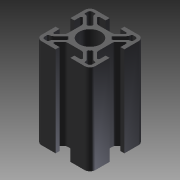
# Autodesk Inventor part: MayTec 1.11.030030.43SP_Profile 30x30. 4F, SP_50_Detail_(0;0,0,0)
Saved by Autodesk Inventor 2011 SP1 (Build 150282100, 282)
## iProperties
Created: 2018-01-06
Part Number: MayTec 1.11.030030.43SP_Profile 30x30. 4F, SP_50_Detail_(0;0,0,0)
Catalog Web Link: www.cadenas.de
Description: 1.11.030030.43SP-Profile 30x30. 4F, SP
Vendor: MAYTEC
Document SubType Name: Modeling
Designer: psAdmin
Manufacturer: MAYTEC
Mass: 18.6034 g
Surface Area: 180.256 cm^2
Volume: 18.6034 cm^3
Density: 1 g/cm^3
Category: PARTsolutions
Company: MAYTEC
Title: MayTec 1.11.030030.43SP_Profile 30x30. 4F, SP_50_Detail_(0;0,0,0)
Author: Cadenas PARTsolutions
Comments: Profile 30x30. 4F, SP
PSOL_IDENT_0: {$CADENAS_DATA\23d-libs\maytec\maytec_3d\profile\profilgruppe_30\30x30\1.11.030030.43sp.prj},299 {VT
PSOL_IDENT_1: YP=3D},{NB=MayTec 1.11.030030.43SP_Profile 30x30. 4F, SP_50_Detail_(0;0,0,0)},{LINA=MayTec 1.11.0300
PSOL_IDENT_2: 30.43SP_Profile 30x30. 4F, SP_50_Detail_(0;0,0,0)},{NN=1.11.030030.43SP},{DATE=09.02.2017 10:28:55},
PSOL_IDENT_3: {GEOMDATE=07.02.2017 11:09:15},{VERSION=},{LINEID=10},{LINESUBID=-1},{WBVAR=L,SAX,SAY,EAX,EAY}  {NB=
PSOL_IDENT_4: MayTec 1.11.030030.43SP_Profile 30x30. 4F, SP_50_Detail_(0;0,0,0)},{LINA=MayTec 1.11.030030.43SP_Pro
PSOL_IDENT_5: file 30x30. 4F, SP_50_Detail_(0;0,0,0)},{KT=DUMMY},{PARTNR=1.11.030030.43SP},{DESCRIPTION=Profil 30x
PSOL_IDENT_6: 30, 4F, SP},{L=50.00},{DETAIL=Detail},{D=1},{XTRANS=Profile 30x30. 4F, SP},{SAX=0},{SAY=0},{EAX=0},{
PSOL_IDENT_7: EAY=0},{BR=30.0},{HE=30.0},{SDX=0},{EDX=0},{MINLENGTHG=1},{MINLENGTH=50}
NN: 1.11.030030.43SP
NT: Profile 30x30. 4F, SP
NB: MayTec 1.11.030030.43SP_Profile 30x30. 4F, SP_50_Detail_(0;0,0,0)
NBSYN: MayTec $PARTNR._$XTRANS._$L._$DETAIL._($SAX.;$SAY.,$EAX.,$EAY.)
LINA: MayTec 1.11.030030.43SP_Profile 30x30. 4F, SP_50_Detail_(0;0,0,0)
PARTNR: 1.11.030030.43SP
DESCRIPTION: Profile 30x30. 4F, SP
L: 50.00
DETAIL: Detail
SUPPLIER: MAYTEC
ARTICLENO: MayTec 1.11.030030.43SP_Profile 30x30. 4F, SP_50_Detail_(0;0,0,0)
BOMINFO: MayTec 1.11.030030.43SP_Profile 30x30. 4F, SP_50_Detail_(0;0,0,0)
CREATOR: CADENAS GmbH
Autodesk Inventor part; units mm, degrees
sketch "Skizze_1" plane through (0, 0, 0) normal (0, 0, 1) x (1, 0, 0)
  line L0 (-15, 4.1) -> (-12.8, 4.1)
  line L1 (-12.8, 4.1) -> (-12.8, 7.3)
  arc A0 (-11.605, 7.795) -> (-12.8, 7.3) centre (-12.1, 7.3) ccw
  line L2 (-11.605, 7.795) -> (-9.0858, 5.2757)
  arc A1 (-8.5, 3.8615) -> (-9.0858, 5.2757) centre (-10.5, 3.8615) ccw
  line L3 (-8.5, 3.8615) -> (-8.5, -3.8615)
  arc A2 (-9.0858, -5.2757) -> (-8.5, -3.8615) centre (-10.5, -3.8615) ccw
  line L4 (-9.0858, -5.2757) -> (-11.605, -7.795)
  arc A3 (-12.8, -7.3) -> (-11.605, -7.795) centre (-12.1, -7.3) ccw
  line L5 (-12.8, -7.3) -> (-12.8, -4.1)
  line L6 (-12.8, -4.1) -> (-15, -4.1)
  line L7 (-15, -4.1) -> (-15, -12)
  arc A4 (-15, -12) -> (-12, -15) centre (-12, -12) ccw
  line L8 (-12, -15) -> (-4.1, -15)
  line L9 (-4.1, -15) -> (-4.1, -12.8)
  line L10 (-4.1, -12.8) -> (-7.3, -12.8)
  arc A5 (-7.795, -11.605) -> (-7.3, -12.8) centre (-7.3, -12.1) ccw
  line L11 (-7.795, -11.605) -> (-5.2757, -9.0858)
  arc A6 (-3.8615, -8.5) -> (-5.2757, -9.0858) centre (-3.8615, -10.5) ccw
  line L12 (-3.8615, -8.5) -> (3.8615, -8.5)
  arc A7 (5.2757, -9.0858) -> (3.8615, -8.5) centre (3.8615, -10.5) ccw
  line L13 (5.2757, -9.0858) -> (7.795, -11.605)
  arc A8 (7.3, -12.8) -> (7.795, -11.605) centre (7.3, -12.1) ccw
  line L14 (7.3, -12.8) -> (4.1, -12.8)
  line L15 (4.1, -12.8) -> (4.1, -15)
  line L16 (4.1, -15) -> (12, -15)
  arc A9 (12, -15) -> (15, -12) centre (12, -12) ccw
  line L17 (15, -12) -> (15, -4.1)
  line L18 (15, -4.1) -> (12.8, -4.1)
  line L19 (12.8, -4.1) -> (12.8, -7.3)
  arc A10 (11.605, -7.795) -> (12.8, -7.3) centre (12.1, -7.3) ccw
  line L20 (11.605, -7.795) -> (9.0858, -5.2757)
  arc A11 (8.5, -3.8615) -> (9.0858, -5.2757) centre (10.5, -3.8615) ccw
  line L21 (8.5, -3.8615) -> (8.5, 3.8615)
  arc A12 (9.0858, 5.2757) -> (8.5, 3.8615) centre (10.5, 3.8615) ccw
  line L22 (9.0858, 5.2757) -> (11.605, 7.795)
  arc A13 (12.8, 7.3) -> (11.605, 7.795) centre (12.1, 7.3) ccw
  line L23 (12.8, 7.3) -> (12.8, 4.1)
  line L24 (12.8, 4.1) -> (15, 4.1)
  line L25 (15, 4.1) -> (15, 12)
  arc A14 (15, 12) -> (12, 15) centre (12, 12) ccw
  line L26 (12, 15) -> (4.1, 15)
  line L27 (4.1, 15) -> (4.1, 12.8)
  line L28 (4.1, 12.8) -> (7.3, 12.8)
  arc A15 (7.795, 11.605) -> (7.3, 12.8) centre (7.3, 12.1) ccw
  line L29 (7.795, 11.605) -> (5.2757, 9.0858)
  arc A16 (3.8615, 8.5) -> (5.2757, 9.0858) centre (3.8615, 10.5) ccw
  line L30 (3.8615, 8.5) -> (-3.8615, 8.5)
  arc A17 (-5.2757, 9.0858) -> (-3.8615, 8.5) centre (-3.8615, 10.5) ccw
  line L31 (-5.2757, 9.0858) -> (-7.795, 11.605)
  arc A18 (-7.3, 12.8) -> (-7.795, 11.605) centre (-7.3, 12.1) ccw
  line L32 (-7.3, 12.8) -> (-4.1, 12.8)
  line L33 (-4.1, 12.8) -> (-4.1, 15)
  line L34 (-4.1, 15) -> (-12, 15)
  arc A19 (-12, 15) -> (-15, 12) centre (-12, 12) ccw
  line L35 (-15, 12) -> (-15, 4.1)
  arc A20 (5.4886, -6.4904) -> (5.4579, -7.2257) centre (5.8115, -6.8722) ccw
  line L36 (5.4579, -7.2257) -> (9.2678, -11.0355)
  arc A21 (10, -12.8006) -> (9.2678, -11.0355) centre (7.5, -12.8033) ccw
  arc A22 (10, -12.8006) -> (10.5, -13.3) centre (10.5, -12.8) ccw
  line L37 (10.5, -13.3) -> (12, -13.3)
  arc A23 (12, -13.3) -> (13.3, -12) centre (12, -12) ccw
  line L38 (13.3, -12) -> (13.3, -10.5)
  arc A24 (13.3, -10.5) -> (12.8006, -10) centre (12.8, -10.5) ccw
  arc A25 (11.0355, -9.2678) -> (12.8006, -10) centre (12.8033, -7.5) ccw
  line L39 (11.0355, -9.2678) -> (7.2257, -5.4579)
  arc A26 (7.2257, -5.4579) -> (6.4904, -5.4886) centre (6.8722, -5.8115) ccw
  arc A27 (5.4886, -6.4904) -> (6.4904, -5.4886) centre (0, 0) ccw
  arc A28 (5.4579, 7.2257) -> (5.4886, 6.4904) centre (5.8115, 6.8722) ccw
  arc A29 (6.4904, 5.4886) -> (5.4886, 6.4904) centre (0, 0) ccw
  arc A30 (6.4904, 5.4886) -> (7.2257, 5.4579) centre (6.8722, 5.8115) ccw
  line L40 (7.2257, 5.4579) -> (11.0355, 9.2678)
  arc A31 (12.8006, 10) -> (11.0355, 9.2678) centre (12.8033, 7.5) ccw
  arc A32 (12.8006, 10) -> (13.3, 10.5) centre (12.8, 10.5) ccw
  line L41 (13.3, 10.5) -> (13.3, 12)
  arc A33 (13.3, 12) -> (12, 13.3) centre (12, 12) ccw
  line L42 (12, 13.3) -> (10.5, 13.3)
  arc A34 (10.5, 13.3) -> (10, 12.8006) centre (10.5, 12.8) ccw
  arc A35 (9.2678, 11.0355) -> (10, 12.8006) centre (7.5, 12.8033) ccw
  line L43 (9.2678, 11.0355) -> (5.4579, 7.2257)
  circle A36 centre (0, 0) radius 6
  line L44 (-13.3, 12) -> (-13.3, 10.5)
  arc A37 (-13.3, 10.5) -> (-12.8006, 10) centre (-12.8, 10.5) ccw
  arc A38 (-11.0355, 9.2678) -> (-12.8006, 10) centre (-12.8033, 7.5) ccw
  line L45 (-11.0355, 9.2678) -> (-7.2257, 5.4579)
  arc A39 (-7.2257, 5.4579) -> (-6.4904, 5.4886) centre (-6.8722, 5.8115) ccw
  arc A40 (-5.4886, 6.4904) -> (-6.4904, 5.4886) centre (0, 0) ccw
  arc A41 (-5.4886, 6.4904) -> (-5.4579, 7.2257) centre (-5.8115, 6.8722) ccw
  line L46 (-5.4579, 7.2257) -> (-9.2678, 11.0355)
  arc A42 (-10, 12.8006) -> (-9.2678, 11.0355) centre (-7.5, 12.8033) ccw
  arc A43 (-10, 12.8006) -> (-10.5, 13.3) centre (-10.5, 12.8) ccw
  line L47 (-10.5, 13.3) -> (-12, 13.3)
  arc A44 (-12, 13.3) -> (-13.3, 12) centre (-12, 12) ccw
  line L48 (-13.3, -10.5) -> (-13.3, -12)
  arc A45 (-13.3, -12) -> (-12, -13.3) centre (-12, -12) ccw
  line L49 (-12, -13.3) -> (-10.5, -13.3)
  arc A46 (-10.5, -13.3) -> (-10, -12.8006) centre (-10.5, -12.8) ccw
  arc A47 (-9.2678, -11.0355) -> (-10, -12.8006) centre (-7.5, -12.8033) ccw
  line L50 (-9.2678, -11.0355) -> (-5.4579, -7.2257)
  arc A48 (-5.4579, -7.2257) -> (-5.4886, -6.4904) centre (-5.8115, -6.8722) ccw
  arc A49 (-6.4904, -5.4886) -> (-5.4886, -6.4904) centre (0, 0) ccw
  arc A50 (-6.4904, -5.4886) -> (-7.2257, -5.4579) centre (-6.8722, -5.8115) ccw
  line L51 (-7.2257, -5.4579) -> (-11.0355, -9.2678)
  arc A51 (-12.8006, -10) -> (-11.0355, -9.2678) centre (-12.8033, -7.5) ccw
  arc A52 (-12.8006, -10) -> (-13.3, -10.5) centre (-12.8, -10.5) ccw
  constraints: 104 end point, 104 point on circle, 53 centre point
extrude "Extrusion1" add sketch "Skizze_1" against normal blind 50
ref_plane "end_XY" through (0, 0, -50) normal (0, 0, -1) x (1, 0, 0)
ref_plane "end_YZ" through (0, 0, -50) normal (1, 0, 0) x (0, -1, 0)
ref_plane "end_ZX" through (0, 0, -50) normal (0, -1, 0) x (0, 0, -1)
ref_plane "side_1a_XY" through (0, 15, -25) normal (0, 1, 0) x (1, 0, 0)
ref_plane "side_1a_YZ" through (0, 15, -25) normal (1, 0, 0) x (0, 0, -1)
ref_plane "side_1a_ZX" through (0, 15, -25) normal (0, 0, -1) x (0, 1, 0)
ref_plane "side_2b_XY" through (15, 0, -25) normal (1, 0, 0) x (0, -1, 0)
ref_plane "side_2b_YZ" through (15, 0, -25) normal (0, -1, 0) x (0, 0, -1)
ref_plane "side_2b_ZX" through (15, 0, -25) normal (0, 0, -1) x (1, 0, 0)
ref_plane "side_3c_XY" through (0, -15, -25) normal (0, -1, 0) x (-1, 0, 0)
ref_plane "side_3c_YZ" through (0, -15, -25) normal (-1, 0, 0) x (0, 0, -1)
ref_plane "side_3c_ZX" through (0, -15, -25) normal (0, 0, -1) x (0, -1, 0)
ref_plane "side_4d_XY" through (-15, 0, -25) normal (-1, 0, 0) x (0, 1, 0)
ref_plane "side_4d_YZ" through (-15, 0, -25) normal (0, 1, 0) x (0, 0, -1)
ref_plane "side_4d_ZX" through (-15, 0, -25) normal (0, 0, -1) x (-1, 0, 0)
ref_plane "start_XY" through (0, 0, 0) normal (0, 0, 1) x (1, 0, 0)
ref_plane "start_YZ" through (0, 0, 0) normal (1, 0, 0) x (0, 1, 0)
ref_plane "start_ZX" through (0, 0, 0) normal (0, 1, 0) x (0, 0, 1)
body "Solid1"
